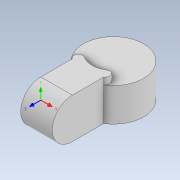
# Autodesk Inventor part: thigh_inventor
Saved by Autodesk Inventor 2020 (Build 240168000, 168)
## iProperties
Created: 2021-01-07
Part Number: thigh_inventor
Material: Generic
Document SubType Name: Modeling
Designer: DELL
Density: 1 g/cm^3
Appearance: Default
Author: DELL
Autodesk Inventor part; units mm, degrees
ref_plane "YZ Plane" through (0, 0, 0) normal (1, 0, 0) x (0, 1, 0)
ref_plane "XZ Plane" through (0, 0, 0) normal (0, 1, 0) x (-1, 0, 0)
ref_plane "XY Plane" through (0, 0, 0) normal (0, 0, 1) x (1, 0, 0)
sketch "Sketch1" plane through (0, 0, 0) normal (0, 1, 0) x (-1, 0, 0)
  line L0 (0, 0) -> (-41.5, 0)
  line L1 (-41.5, 0) -> (-41.5, -75)
  line L2 (-41.5, -75) -> (0, -75)
  line L3 (0, -75) -> (0, 0)
  circle A0 centre (-20.75, -75) radius 39.5
  point P0 (-41.5, -41.3892)
  point P1 (0, -41.3892)
  dimension "d0" = 41.5
  dimension "d1" = 79
  dimension "d14" = 75
  constraints: 8 end point, 2 parallel, 1 centre point, 1 horizontal, 1 midpoint, 1 perpendicular
  measures "d0" distance between parallel lines of L1 L3
  measures "d1" diameter of A0
  measures "d14" distance between parallel lines of L0 L2
extrude "Extrusion1" add sketch "Sketch1" along normal mid plane 53
sketch "Sketch2" plane through (0, 0, 0) normal (1, 0, 0) x (0, 1, 0)
  line L0 (-26.5, 0) -> (26.5, 0) projected
  circle A0 centre (0, 0) radius 26.5
  constraints: 1 midpoint, 3 other
extrude "Extrusion2" add sketch "Sketch2" along normal up to surface (41.5 mm away) contours A0 L0 picked at (8.0782, 6.219)
sketch "Sketch3" plane through (0, 26.5, 0) normal (0, 1, 0) x (1, 0, 0)
  arc A0 (41.5, 41.3892) -> (0, 41.3892) centre (20.75, 75) ccw projected
  circle A1 centre (20.75, 75) radius 39.5
  circle A2 centre (20.75, 75) radius 28
  line L0 (0, -26.5) -> (41.5, -26.5) construction
  line L1 (20.75, -26.5) -> (20.75, 75) construction
  circle A3 centre (38.6348, 46.3784) radius 5.75
  circle A4 centre (2.8652, 46.3784) radius 5.75
  line L2 (20.75, 75) -> (38.6348, 46.3784) construction
  line L3 (2.8652, 46.3784) -> (20.7725, 75.0361) construction
  line L4 (41.5, 41.3892) -> (41.5, 41.3931)
  line L5 (0, 41.3892) -> (0, 0) projected
  line L6 (0, 41.3892) -> (0, 41.3931)
  point P0 (-0.1818, 41.5021)
  point P1 (5.9123, 51.2547)
  point P2 (35.5877, 51.2547)
  point P3 (41.6818, 41.5021)
  point P4 (0, 41.3892)
  point P5 (41.6818, 41.5021)
  point P6 (60.25, 75)
  point P7 (-0.1818, 41.5021)
  point P8 (35.5877, 51.2547)
  dimension "d15" = 56
  dimension "d16" = 32
  constraints: 10 end point, 2 coincident, 2 vertical, 1 centre point, 1 collinear, 1 midpoint, 14 other
  measures "d15" diameter of A2
  measures "d16" angle of L1 L2
extrude "Extrusion3" cut sketch "Sketch3" against normal blind 9 contours L4 A3 A0 | A3 A2 A4 A0 | A0 A4 L6 | A2
body "Solid1"
